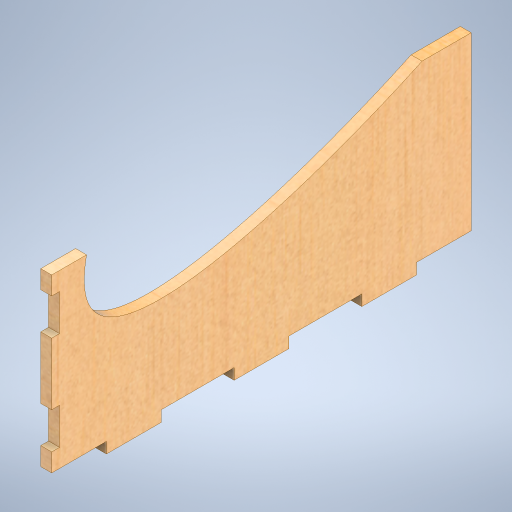
# Autodesk Inventor part: бок
Saved by Autodesk Inventor 2024.2 (Build 282272000, 272)
## iProperties
Created: 2026-01-28
Part Number: бок
Material: Типовые
Document SubType Name: Modeling
Designer: Zakhar
Density: 1 g/cm^3
Appearance: Желтая сосна — массив — светлое морение — со слабым глянцем
Author: Zakhar
Autodesk Inventor part; units mm, degrees
ref_plane "YZ Plane" through (0, 0, 0) normal (1, 0, 0) x (0, 1, 0)
ref_plane "XZ Plane" through (0, 0, 0) normal (0, 1, 0) x (-1, 0, 0)
ref_plane "XY Plane" through (0, 0, 0) normal (0, 0, 1) x (1, 0, 0)
sketch "Эскиз1" plane through (0, 0, 0) normal (1, 0, 0) x (0, 1, 0)
  line L0 (35.7991, 101.2153) -> (-64.2009, 101.2153)
  line L1 (-64.2009, 101.2153) -> (-64.2009, -128.7847)
  line L2 (-64.2009, -128.7847) -> (35.7991, -128.7847)
  line L3 (35.7991, -128.7847) -> (35.7991, 101.2153)
  spline S0 degree 3 poles (35.7991, 82.11) (-39.3429, 97.9126) (5.4102, -36.8519) (35.7991, -101.803) knots 0 0 0 0 1 1 1 1
  point P0 (0, 0)
  point P1 (-0.0002, 69.5079)
  dimension "d0" = 230
  dimension "d1" = 100
  constraints: 8 end point, 2 parallel, 2 point on line, 1 horizontal, 1 perpendicular, 4 other
  measures "d0" distance of L0.end L1.end
  measures "d1" distance of L0.start L0.end
extrude "Выдавливание1" add sketch "Эскиз1" along normal blind 6 contours L3 S0 L2 L1 L0
sketch "Эскиз2" plane through (6, 0, 0) normal (1, 0, 0) x (0, 0, -1)
  line L0 (-101.2153, 35.7991) -> (-101.2153, -64.2009) projected
  line L1 (-101.2153, -64.2009) -> (128.7847, -64.2009) projected
  line L2 (-101.2153, -58.2009) -> (-71.2153, -58.2009)
  line L3 (-71.2153, -58.2009) -> (-71.2153, -64.2009)
  line L4 (-71.2153, -64.2009) -> (-101.2153, -64.2009)
  line L5 (-101.2153, -64.2009) -> (-101.2153, -58.2009)
  line L6 (-71.2153, -58.2009) -> (-41.2153, -58.2009)
  line L7 (-41.2153, -58.2009) -> (-41.2153, -64.2009)
  line L8 (-41.2153, -64.2009) -> (-71.2153, -64.2009)
  line L9 (-71.2153, -64.2009) -> (-71.2153, -58.2009)
  line L10 (-41.2153, -58.2009) -> (-1.2153, -58.2009)
  line L11 (-1.2153, -58.2009) -> (-1.2153, -64.2009)
  line L12 (-1.2153, -64.2009) -> (-41.2153, -64.2009)
  line L13 (-41.2153, -64.2009) -> (-41.2153, -58.2009)
  line L14 (128.7847, -64.2009) -> (128.7847, 35.7991) projected
  line L15 (128.7847, -58.2009) -> (98.7847, -58.2009)
  line L16 (98.7847, -58.2009) -> (98.7847, -64.2009)
  line L17 (98.7847, -64.2009) -> (128.7847, -64.2009)
  line L18 (128.7847, -64.2009) -> (128.7847, -58.2009)
  line L19 (98.7847, -58.2009) -> (68.7847, -58.2009)
  line L20 (68.7847, -58.2009) -> (68.7847, -64.2009)
  line L21 (68.7847, -64.2009) -> (98.7847, -64.2009)
  line L22 (98.7847, -64.2009) -> (98.7847, -58.2009)
  line L23 (68.7847, -58.2009) -> (28.7847, -58.2009)
  line L24 (28.7847, -58.2009) -> (28.7847, -64.2009)
  line L25 (28.7847, -64.2009) -> (68.7847, -64.2009)
  line L26 (68.7847, -64.2009) -> (68.7847, -58.2009)
  line L27 (28.7847, -58.2009) -> (-1.2153, -58.2009)
  line L28 (-1.2153, -58.2009) -> (-1.2153, -64.2009)
  line L29 (-1.2153, -64.2009) -> (28.7847, -64.2009)
  line L30 (28.7847, -64.2009) -> (28.7847, -58.2009)
  point P0 (0, 0)
  dimension "d4" = 30
  dimension "d5" = 30
  dimension "d6" = 40
  dimension "d7" = 30
  dimension "d8" = 30
  dimension "d9" = 40
  dimension "d12" = 6
  dimension "d13" = 6
  constraints: 56 end point, 14 parallel, 8 point on line, 7 horizontal, 7 perpendicular
  measures "d4" distance of L2.start L2.end
  measures "d5" distance of L2.end L6.end
  measures "d6" distance of L6.end L10.end
  measures "d7" distance of L15.start L15.end
  measures "d8" distance of L15.end L19.end
  measures "d9" distance of L19.end L23.end
  measures "d12" distance of L2.end L3.end
  measures "d13" distance of L27.end L11.end
extrude "Выдавливание2" cut sketch "Эскиз2" against normal through all contours L2 L3 L1 L0 | L10 L11 L1 L7 | L23 L20 L1 L24 | L15 L14 L1 L16
sketch "Эскиз3" plane through (0, 0, 0) normal (-1, 0, 0) x (0, 0, 1)
  line L0 (101.2153, -58.2009) -> (96.9434, -58.2009)
  line L1 (96.9434, -58.2009) -> (96.9434, -48.2009)
  line L2 (96.9434, -48.2009) -> (101.2153, -48.2009)
  line L3 (101.2153, -48.2009) -> (101.2153, -58.2009)
  line L4 (96.9434, -48.2009) -> (101.2153, -48.2009)
  line L5 (101.2153, -48.2009) -> (101.2153, -28.2009)
  line L6 (101.2153, -28.2009) -> (96.9434, -28.2009)
  line L7 (96.9434, -28.2009) -> (96.9434, -48.2009)
  line L8 (101.2153, -28.2009) -> (96.9434, -28.2009)
  line L9 (96.9434, -28.2009) -> (96.9434, 5.7991)
  line L10 (96.9434, 5.7991) -> (101.2153, 5.7991)
  line L11 (101.2153, 5.7991) -> (101.2153, -28.2009)
  line L12 (96.9434, 5.7991) -> (101.2153, 5.7991)
  line L13 (101.2153, 5.7991) -> (101.2153, 25.7991)
  line L14 (101.2153, 25.7991) -> (96.9434, 25.7991)
  line L15 (96.9434, 25.7991) -> (96.9434, 5.7991)
  line L16 (101.2153, 35.7991) -> (101.2153, -58.2009) projected
  line L17 (96.9434, 25.7991) -> (101.2153, 25.7991)
  line L18 (101.2153, 25.7991) -> (101.2153, 35.7991)
  line L19 (101.2153, 35.7991) -> (96.9434, 35.7991)
  line L20 (96.9434, 35.7991) -> (96.9434, 25.7991)
  point P0 (0, 0)
  dimension "d14" = 10
  dimension "d15" = 10
  dimension "d16" = 20
  dimension "d17" = 20
  constraints: 40 end point, 10 parallel, 5 horizontal, 5 perpendicular, 3 point on line
  measures "d14" distance of L0.end L1.end
  measures "d15" distance of L19.end L14.end
  measures "d16" distance of L6.end L1.end
  measures "d17" distance of L14.end L9.end
extrude "Выдавливание3" cut sketch "Эскиз3" against normal blind 6 contours L2 L7 L6 L5 | L10 L15 L14 L13
